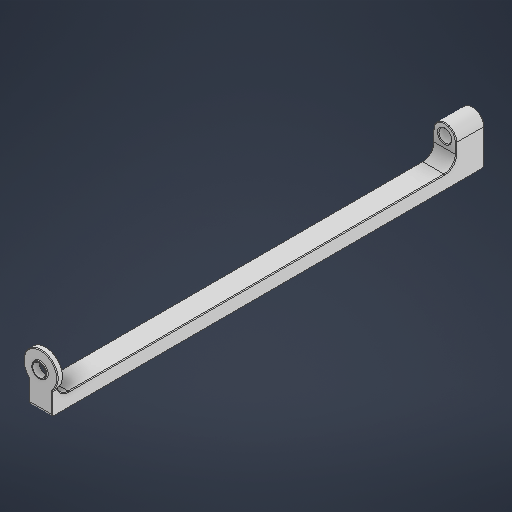
# Autodesk Inventor part: Half-Shaft-Motor
Saved by Autodesk Inventor 2025 (Build 290162010, 162A)
## iProperties
Created: 2025-12-05
Part Number: Half-Shaft-Motor
Material: Generic
Document SubType Name: Modeling
Designer: FizzyApple12
Density: 1 g/cm^3
Appearance: Default
Author: FizzyApple12
Autodesk Inventor part; units mm, degrees
ref_plane "YZ Plane" through (0, 0, 0) normal (1, 0, 0) x (0, 1, 0)
ref_plane "XZ Plane" through (0, 0, 0) normal (0, 1, 0) x (-1, 0, 0)
ref_plane "XY Plane" through (0, 0, 0) normal (0, 0, 1) x (1, 0, 0)
sketch "Sketch1" plane through (0, 0, 0) normal (0, 0, 1) x (1, 0, 0)
  circle A0 centre (0, 0) radius 2.5
  line L0 (-4, -7.6487) -> (4, -7.6487)
  line L1 (4, -7.6487) -> (4, -12.6487)
  line L2 (4, -12.6487) -> (-4, -12.6487)
  line L3 (-4, -12.6487) -> (-4, -7.6487)
  line L4 (0, 0) -> (0, -7.6487) construction
  line L5 (-4, -7.6487) -> (4, -7.6487)
  line L6 (4, -7.6487) -> (4, 4)
  line L7 (4, 4) -> (-4, 4)
  line L8 (-4, 4) -> (-4, -7.6487)
  line L9 (0, 0) -> (0, 4) construction
  line L10 (-4, 4) -> (4, 4)
  line L11 (4, 4) -> (4, 8.5)
  line L12 (4, 8.5) -> (-4, 8.5)
  line L13 (-4, 8.5) -> (-4, 4)
  circle A1 centre (0, 0) radius 6
  circle A2 centre (0, 0) radius 2.2
  point P0 (0, 2.5)
  point P1 (-4, -4.4721)
  point P2 (4, -4.4721)
  dimension "d0" = 5
  dimension "d1" = 8
  dimension "d2" = 5
  dimension "d3" = 4
  dimension "d18" = 6
  dimension "d37" = 12
  dimension "d38" = 4.4
  constraints: 28 end point, 6 parallel, 4 coincident, 3 horizontal, 3 perpendicular, 2 centre point, 2 midpoint, 1 point on line, 1 vertical, 1 vertical alignment, 2 other
  measures "d1" distance of L1.end L2.end
  measures "d2" distance of L0.end L1.end
  measures "d3" distance of L4.start L9.end
  measures "d18" distance from line of L12 point (0, 2.5)
  measures "d37" diameter of A1
  measures "d38" diameter of A2
extrude "Extrusion1" add sketch "Sketch1" against normal blind 2 contours A0 | L8 A1 L6 L0 | L0 L1 L2 L3 | A1 L13 L8 | L8 L7 L6 A1 | L6 L11 A1 | L13 A1 L11 L7 | A2
extrude "Extrusion2" add sketch "Sketch1" against normal blind 152.3335 contours L0 L1 L2 L3
extrude "Extrusion3" add sketch "Sketch1" along normal blind 10 from surface at -152.3335 contours A0 | L8 A1 L6 L0 | L0 L1 L2 L3 | L8 L7 L6 A1 | A2
sketch "Sketch2" plane through (0, 0, -152.3335) normal (0, 0, -1) x (-1, 0, 0)
  point P0 (0, 0)
  point P1 (0, 0)
hole "Hole1" at (0, 0, -152.3335) direction (0, 0, 1) diameter 4.5 depth 12 tip angle 118
hole "Hole3" at (0, 0, 0) direction (0, 0, -1) diameter 4.4 depth 12 tip angle 118
extrude "Extrusion4" add sketch "Sketch1" along normal blind 0.5 contours A0
fillet "Fillet1" radius 4 4 edges at (4, 4, -147.3335) (-4, 4, -147.3335) (0, -7.6487, -2) (0, -7.6487, -142.3335)
fillet "Fillet2" radius 1 4 edges at (0, -12.6487, 0) (0, -12.6487, -152.3335) (-4, -4.4721, -1.0428) (4, -4.4721, -1.0428)
chamfer "Chamfer1" distance 0.25 angle 45 36 edges at (-2.8285, 2.8285, -152.3335) (0, 4, -152.3335) (2.8285, 2.8285, -152.3335) (-4, -5.8243, -152.3335) (-4, -12.3558, -152.0406) (-4, -12.6487, -76.1667) (-4, -12.3558, -0.2929) (-4, -8.2738, 0) (-4.0742, -4.521, 0) (0, 6, 0) (4.0742, -4.521, 0) (4, -8.2738, 0) (4, -12.3558, -0.2929) (4, -12.6487, -76.1667) (4, -12.3558, -152.0406) (4, -5.8243, -152.3335) (0, -2.25, -152.3335) (0, -2.25, -142.3335) (-2.8285, 2.8285, -142.3335) (0, 4, -142.3335) (2.8285, 2.8285, -142.3335) (4, -1.8244, -142.3335) (4, -6.4772, -141.162) (4, -7.6487, -72.1667) (4, -6.8892, -3.6548) (4.0764, -4.5156, -2.095) (4.5301, -3.9343, -2.0102) (0, 6, -2) (-4.5299, -3.9344, -2.0102) (-4.0764, -4.5157, -2.0951) (-4, -6.8892, -3.6548) (-4, -7.6487, -72.1667) (-4, -6.4772, -141.162) (-4, -1.8244, -142.3335) (0, 2.2, -2) (-2.5, 0, 0)
body "Solid1"
